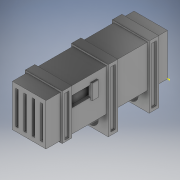
# Autodesk Inventor part: Part1
Saved by Autodesk Inventor 2021 (Build 250183000, 183)
## iProperties
Created: 2021-05-04
Part Number: Part1
Material: Generic
Document SubType Name: Modeling
Designer: AHUJA
Density: 1 g/cm^3
Appearance: Default
Author: AHUJA
Autodesk Inventor part; units mm, degrees
(part 1 of 2)
ref_plane "YZ Plane" through (0, 0, 0) normal (1, 0, 0) x (0, 1, 0)
ref_plane "XZ Plane" through (0, 0, 0) normal (0, 1, 0) x (-1, 0, 0)
sketch "Sketch1" plane through (0, 0, 0) normal (0, 0, 1) x (1, 0, 0)
  line L0 (0, 0) -> (50.8, 0)
  line L1 (50.8, 0) -> (50.8, 63.5)
  line L2 (50.8, 63.5) -> (0, 63.5)
  line L3 (0, 63.5) -> (0, 0)
  dimension "d0" = 63.5
  dimension "d1" = 50.8
  constraints: 8 end point, 2 parallel, 1 horizontal, 1 perpendicular
  measures "d0" distance of L0.end L1.end
  measures "d1" distance of L1.end L2.end
extrude "Extrusion1" add sketch "Sketch1" along normal blind 184.15
sketch "Sketch2" plane through (0, 0, 184.15) normal (0, 0, 1) x (1, 0, 0)
  line L0 (5.021, 56.896) -> (8.763, 56.896)
  line L1 (8.763, 56.896) -> (8.763, 6.604)
  line L2 (8.763, 6.604) -> (5.021, 6.604)
  line L3 (5.021, 6.604) -> (5.021, 56.896)
  line L4 (0, 63.5) -> (0, 0) projected
  line L5 (50.8, 63.5) -> (0, 63.5) projected
  line L6 (17.467, 56.896) -> (21.209, 56.896)
  line L7 (21.209, 56.896) -> (21.209, 6.604)
  line L8 (21.209, 6.604) -> (17.467, 6.604)
  line L9 (17.467, 6.604) -> (17.467, 56.896)
  line L10 (29.913, 56.896) -> (33.655, 56.896)
  line L11 (33.655, 56.896) -> (33.655, 6.604)
  line L12 (33.655, 6.604) -> (29.913, 6.604)
  line L13 (29.913, 6.604) -> (29.913, 56.896)
  line L14 (42.359, 56.896) -> (46.101, 56.896)
  line L15 (46.101, 56.896) -> (46.101, 6.604)
  line L16 (46.101, 6.604) -> (42.359, 6.604)
  line L17 (42.359, 6.604) -> (42.359, 56.896)
  line L18 (50.8, 0) -> (50.8, 63.5) projected
  dimension "d4" = 3.742
  dimension "d5" = 50.292
  dimension "d6" = 5.021
  dimension "d7" = 6.604
  dimension "d8" = 8.704
  dimension "d9" = 6.604
  dimension "d10" = 3.742
  dimension "d11" = 3.742
  dimension "d12" = 8.704
  dimension "d13" = 3.742
  dimension "d16" = 8.704
  constraints: 32 end point, 8 parallel, 4 horizontal, 4 perpendicular
  measures "d4" distance of L0.start L0.end
  measures "d5" distance of L0.end L1.end
  measures "d6" distance between parallel lines of L4 L3
  measures "d7" distance between parallel lines of L5 L0
  measures "d8" distance between parallel lines of L1 L9
  measures "d9" distance between parallel lines of L5 L6
  measures "d10" distance of L6.start L6.end
  measures "d11" distance of L10.start L10.end
  measures "d12" distance between parallel lines of L13 L7
  measures "d13" distance of L14.start L14.end
  measures "d16" distance between parallel lines of L17 L11
extrude "Extrusion2" cut sketch "Sketch2" against normal blind 100
sketch "Sketch3" plane through (0, 0, 0) normal (-1, 0, 0) x (0, 0, 1)
  line L0 (15.895, 66.04) -> (30.358, 66.04)
  line L1 (30.358, 66.04) -> (30.358, -28.667)
  line L2 (30.358, -28.667) -> (15.895, -28.667)
  line L3 (15.895, -28.667) -> (15.895, 66.04)
  line L4 (0, 63.5) -> (0, 0) projected
  line L5 (0, 63.5) -> (184.15, 63.5) projected
  line L6 (77.905, 66.04) -> (92.368, 66.04)
  line L7 (92.368, 66.04) -> (92.368, -28.667)
  line L8 (92.368, -28.667) -> (77.905, -28.667)
  line L9 (77.905, -28.667) -> (77.905, 66.04)
  line L10 (147.737, 66.04) -> (162.2, 66.04)
  line L11 (162.2, 66.04) -> (162.2, -2.54)
  line L12 (162.2, -2.54) -> (147.737, -2.54)
  line L13 (147.737, -2.54) -> (147.737, 66.04)
  dimension "d19" = 94.707
  dimension "d20" = 14.463
  dimension "d21" = 15.895
  dimension "d22" = 2.54
  dimension "d23" = 94.707
  dimension "d24" = 14.463
  dimension "d25" = 68.58
  dimension "d26" = 14.463
  dimension "d27" = 2.54
  dimension "d28" = 2.54
  dimension "d29" = 47.547
  dimension "d30" = 55.369
  constraints: 24 end point, 6 parallel, 3 horizontal, 3 perpendicular
  measures "d19" distance of L0.end L1.end
  measures "d20" distance of L0.start L0.end
  measures "d21" distance between parallel lines of L4 L3
  measures "d22" distance between parallel lines of L5 L0
  measures "d23" distance of L6.end L7.end
  measures "d24" distance of L6.start L6.end
  measures "d25" distance of L10.end L11.end
  measures "d26" distance of L10.start L10.end
  measures "d27" distance between parallel lines of L5 L10
  measures "d28" distance between parallel lines of L5 L6
  measures "d29" distance between parallel lines of L9 L1
  measures "d30" distance between parallel lines of L13 L7
ref_plane "Work Plane1" through (53.34, 0, 0) normal (1, 0, 0) x (0, 0, -1)
extrude "Extrusion3" add sketch "Sketch3" along normal blind 55.88 from surface at -53.34
sketch "Sketch4" plane through (-2.54, -28.667, 30.358) normal (-1, 0, 0) x (0, 0, 1)
  point P0 (-30.358, 28.667)
sketch "Sketch5" plane through (-2.54, -28.667, 30.358) normal (-1, 0, 0) x (0, 0, 1)
  line L0 (-10.738, 90.177) -> (-3.756, 90.177)
  line L1 (-3.756, 90.177) -> (-3.756, 4.938)
  line L2 (-3.756, 4.938) -> (-10.738, 4.938)
  line L3 (-10.738, 4.938) -> (-10.738, 90.177)
  line L4 (-14.463, 94.707) -> (-14.463, 0) projected
  line L5 (51.272, 90.177) -> (58.254, 90.177)
  line L6 (58.254, 90.177) -> (58.254, 4.938)
  line L7 (58.254, 4.938) -> (51.272, 4.938)
  line L8 (51.272, 4.938) -> (51.272, 90.177)
  line L9 (47.547, 94.707) -> (47.547, 0) projected
  line L10 (0, 94.707) -> (-14.463, 94.707) projected
  line L11 (62.01, 94.707) -> (47.547, 94.707) projected
  line L12 (121.666, 90.087) -> (127.547, 90.087)
  line L13 (127.547, 90.087) -> (127.547, 28.667)
  line L14 (127.547, 28.667) -> (121.666, 28.667)
  line L15 (121.666, 28.667) -> (121.666, 90.087)
  line L16 (117.379, 94.707) -> (117.379, 26.127) projected
  point P0 (-30.358, 28.667)
  dimension "d34" = 6.982
  dimension "d35" = 85.239
  dimension "d36" = 3.725
  dimension "d37" = 6.982
  dimension "d38" = 85.239
  dimension "d39" = 3.725
  dimension "d40" = 4.53
  dimension "d41" = 4.53
  dimension "d42" = 61.42
  dimension "d43" = 5.881
  dimension "d44" = 4.287
  constraints: 24 end point, 6 parallel, 3 horizontal, 3 perpendicular
  measures "d34" distance of L0.start L0.end
  measures "d35" distance of L0.end L1.end
  measures "d36" distance between parallel lines of L4 L3
  measures "d37" distance of L5.start L5.end
  measures "d38" distance of L5.end L6.end
  measures "d39" distance between parallel lines of L9 L8
  measures "d40" distance between parallel lines of L10 L0
  measures "d41" distance between parallel lines of L11 L5
  measures "d42" distance of L12.end L13.end
  measures "d43" distance of L12.start L12.end
  measures "d44" distance between parallel lines of L16 L15
extrude "Extrusion4" cut sketch "Sketch5" against normal blind 2.54
sketch "Sketch6" plane through (0, 0, 92.368) normal (-1, 0, 0) x (0, 0, 1)
  line L0 (14.937, 53.681) -> (24.354, 53.681)
  line L1 (24.354, 53.681) -> (24.354, 30.706)
  line L2 (24.354, 30.706) -> (14.937, 30.706)
  line L3 (14.937, 30.706) -> (14.937, 53.681)
  line L4 (0, -28.667) -> (0, 66.04) projected
  line L5 (0, 63.5) -> (55.369, 63.5) projected
  point P0 (-92.368, 0)
  dimension "d48" = 9.417
  dimension "d49" = 14.937
  dimension "d50" = 9.819
  dimension "d51" = 22.975
  constraints: 8 end point, 2 parallel, 1 horizontal, 1 perpendicular
  measures "d48" distance of L0.start L0.end
  measures "d49" distance between parallel lines of L4 L3
  measures "d50" distance between parallel lines of L5 L0
  measures "d51" distance of L2.end L0.start
extrude "Extrusion5" add sketch "Sketch6" along normal blind 1.905
sketch "Sketch7" plane through (0, 0, 92.368) normal (-1, 0, 0) x (0, 0, 1)
  line L0 (24.354, 30.706) -> (24.354, 53.681) projected
  line L1 (24.354, 50.479) -> (55.5483, 50.479)
  line L2 (55.5483, 50.479) -> (55.5483, 34.348)
  line L3 (55.5483, 34.348) -> (24.354, 34.348)
  line L4 (24.354, 34.348) -> (24.354, 50.479)
  line L5 (0, 63.5) -> (55.369, 63.5) projected
  point P0 (-92.368, 0)
  dimension "d54" = 13.021
  dimension "d55" = 16.131
  constraints: 8 end point, 2 parallel, 1 horizontal, 1 perpendicular, 1 point on line
  measures "d54" distance between parallel lines of L5 L1
  measures "d55" distance of L1.end L2.end
extrude "Extrusion6" cut sketch "Sketch7" against normal blind 6.926
sketch "Sketch8" plane through (-1.905, 53.681, 116.722) normal (0, 0, 1) x (1, 0, 0)
  point P0 (1.905, -53.681)
sketch "Sketch9" plane through (-1.905, 53.681, 116.722) normal (0, 0, 1) x (1, 0, 0)
  line L0 (1.905, -19.333) -> (6.926, -19.333) projected
  line L1 (6.926, -19.333) -> (5.021, -19.333)
  line L2 (5.021, -19.333) -> (5.021, -3.202)
  line L3 (5.021, -3.202) -> (6.926, -3.202)
  line L4 (6.926, -3.202) -> (6.926, -19.333)
  point P0 (1.905, -53.681)
  dimension "d58" = 16.131
  dimension "d59" = 1.905
  constraints: 8 end point, 2 parallel, 1 horizontal, 1 perpendicular
  measures "d58" distance of L1.end L2.end
  measures "d59" distance of L0.end L1.end
extrude "Extrusion7" cut sketch "Sketch9" against normal blind 9.417
sketch "Sketch10" plane through (53.34, 66.04, 15.895) normal (0, 0, -1) x (-1, 0, 0)
  circle A0 centre (28.738, -80.425) radius 12.0905
  line L0 (55.88, 0) -> (55.88, -94.707) projected
  line L1 (0, -94.707) -> (55.88, -94.707) projected
  point P0 (53.34, -66.04)
  dimension "d62" = 27.142
  dimension "d63" = 14.282
  dimension "d64" = 24.181
  constraints: 1 centre point
  measures "d62" distance from line of L0 A0.centre
  measures "d63" distance from line of L1 A0.centre
  measures "d64" diameter of A0
sketch "Sketch11" plane through (53.34, 66.04, 77.905) normal (0, 0, -1) x (-1, 0, 0)
  circle A0 centre (27.142, -80.425) radius 12.0905
  line L0 (0, -94.707) -> (55.88, -94.707) projected
  line L1 (0, 0) -> (0, -94.707) projected
  point P0 (53.34, -66.04)
  dimension "d65" = 24.181
  dimension "d66" = 14.282
  dimension "d67" = 27.142
  constraints: 1 centre point
  measures "d65" diameter of A0
  measures "d66" distance from line of L0 A0.centre
  measures "d67" distance from line of L1 A0.centre
extrude "Extrusion8" cut sketch "Sketch10" against normal blind 30
extrude "Extrusion9" cut sketch "Sketch11" against normal blind 30
sketch "Sketch12" plane through (0, 0, 0) normal (0, 0, -1) x (-1, 0, 0)
  line L0 (-25.449, 0) -> (-24.765, 0)
  line L1 (-24.765, 0) -> (-24.765, 0.127)
  line L2 (-24.765, 0.127) -> (-25.449, 0.127)
  line L3 (-25.449, 0.127) -> (-25.449, 0)
  line L4 (0, 63.5) -> (0, 0) projected
  dimension "d72" = 0.127
  dimension "d73" = 0.684
  dimension "d74" = 24.765
  constraints: 8 end point, 2 parallel, 1 horizontal, 1 perpendicular
  measures "d72" distance of L0.end L1.end
  measures "d73" distance of L1.end L2.end
  measures "d74" distance between parallel lines of L4 L1
extrude "Extrusion10" cut sketch "Sketch12" against normal blind 500
sketch "Sketch13" plane through (50.8, 0, 92.368) normal (1, 0, 0) x (0, 0, -1)
  point P0 (92.368, 0)
sketch "Sketch14" plane through (50.8, 0, 92.368) normal (1, 0, 0) x (0, 0, -1)
  line L0 (-55.369, 56.896) -> (-55.369, 6.604) projected
  line L1 (-24.354, 50.479) -> (-24.354, 34.348)
  line L2 (-55.369, 34.348) -> (-55.369, 50.479)
  line L3 (0, 63.5) -> (-55.369, 63.5) projected
  line L4 (-14.937, 53.681) -> (-24.354, 53.681)
  line L5 (-24.354, 53.681) -> (-24.354, 30.706)
  line L6 (-24.354, 30.706) -> (-14.937, 30.706)
  line L7 (-14.937, 30.706) -> (-14.937, 53.681)
  point P0 (92.368, 0)
  point P1 (-24.354, 50.479)
  point P2 (-24.354, 34.348)
  dimension "d77" = 31.015
  dimension "d80" = 9.819
  dimension "d81" = 9.417
  dimension "d82" = 22.975
  constraints: 12 end point, 3 parallel, 1 horizontal, 1 perpendicular, 1 point on line
  measures "d77" distance of L2.end L1.start
  measures "d80" distance between parallel lines of L3 L4
  measures "d81" distance of L4.start L4.end
  measures "d82" distance of L6.end L4.start
extrude "Extrusion11" add sketch "Sketch14" along normal mid plane 5.021
sketch "Sketch15" plane through (50.8, 0, 92.368) normal (1, 0, 0) x (0, 0, -1)
  line L0 (-55.369, 63.5) -> (-55.369, 0) projected
  line L1 (-24.354, 53.681) -> (-24.354, 30.706) projected
  line L2 (-55.369, 50.479) -> (-24.354, 50.479)
  line L3 (-24.354, 50.479) -> (-24.354, 34.348)
  line L4 (-24.354, 34.348) -> (-55.369, 34.348)
  line L5 (-55.369, 34.348) -> (-55.369, 50.479)
  line L6 (0, 63.5) -> (-55.369, 63.5) projected
  point P0 (92.368, 0)
  dimension "d85" = 16.131
  dimension "d86" = 13.021
  constraints: 8 end point, 2 parallel, 2 point on line, 1 horizontal, 1 perpendicular
  measures "d85" distance between parallel lines of L4 L2
  measures "d86" distance between parallel lines of L6 L2
extrude "Extrusion12" cut sketch "Sketch15" against normal blind 5.021
sketch "Sketch16" plane through (50.8, 30.706, 116.722) normal (0, 0, 1) x (1, 0, 0)
  line L0 (0, 3.642) -> (-4.699, 3.642) projected
  line L1 (-4.699, 3.642) -> (-2.794, 3.642)
  line L2 (-2.794, 3.642) -> (-2.794, 19.773)
  line L3 (-2.794, 19.773) -> (-4.699, 19.773)
  line L4 (-4.699, 19.773) -> (-4.699, 3.642)
  point P0 (-50.8, -30.706)
  point P1 (-2.794, 3.642)
  dimension "d89" = 16.131
  dimension "d90" = 1.905
  constraints: 8 end point, 2 parallel, 1 horizontal, 1 perpendicular
  measures "d89" distance of L1.end L2.end
  measures "d90" distance of L2.end L3.end
extrude "Extrusion13" cut sketch "Sketch16" against normal blind 9.417
sketch "Sketch17" plane through (50.8, 0, 92.368) normal (0, -1, 0) x (1, 0, 0)
  line L0 (-40.298, 34.057) -> (-10.502, 34.057)
  line L1 (-10.502, 34.057) -> (-10.502, 27.55)
  line L2 (-10.502, 27.55) -> (-40.298, 27.55)
  line L3 (-40.298, 27.55) -> (-40.298, 34.057)
  line L4 (0, 0) -> (0, 55.369) projected
  line L5 (-50.8, 0) -> (-50.8, 55.369) projected
  line L6 (2.54, 55.369) -> (-53.34, 55.369) projected
  line L7 (-40.298, -35.775) -> (-10.502, -35.775)
  line L8 (-10.502, -35.775) -> (-10.502, -42.282)
  line L9 (-10.502, -42.282) -> (-40.298, -42.282)
  line L10 (-40.298, -42.282) -> (-40.298, -35.775)
  line L11 (0, -62.01) -> (0, -14.463) projected
  line L12 (-50.8, -62.01) -> (-50.8, -14.463) projected
  line L13 (2.54, -14.463) -> (-53.34, -14.463) projected
  point P0 (-50.8, -92.368)
  dimension "d93" = 10.502
  dimension "d94" = 10.502
  dimension "d95" = 6.507
  dimension "d96" = 21.312
  dimension "d97" = 6.507
  dimension "d98" = 10.502
  dimension "d99" = 10.502
  dimension "d100" = 21.312
  constraints: 16 end point, 4 parallel, 2 horizontal, 2 perpendicular
  measures "d93" distance between parallel lines of L4 L1
  measures "d94" distance between parallel lines of L5 L3
  measures "d95" distance between parallel lines of L2 L0
  measures "d96" distance between parallel lines of L0 L6
  measures "d97" distance between parallel lines of L9 L7
  measures "d98" distance between parallel lines of L11 L8
  measures "d99" distance between parallel lines of L12 L10
  measures "d100" distance between parallel lines of L13 L7
extrude "Extrusion14" add sketch "Sketch17" along normal blind 2.54
sketch "Sketch18" plane through (53.34, -2.54, 147.737) normal (1, 0, 0) x (0, 0, -1)
  point P0 (147.737, 2.54)
sketch "Sketch19" plane through (53.34, -2.54, 147.737) normal (1, 0, 0) x (0, 0, -1)
  point P0 (147.737, 2.54)
sketch "Sketch20" plane through (53.34, -2.54, 147.737) normal (1, 0, 0) x (0, 0, -1)
  line L0 (-10.168, 63.96) -> (-4.287, 63.96)
  line L1 (-4.287, 63.96) -> (-4.287, 2.54)
  line L2 (-4.287, 2.54) -> (-10.168, 2.54)
  line L3 (-10.168, 2.54) -> (-10.168, 63.96)
  line L4 (-14.463, 68.58) -> (0, 68.58) projected
  line L5 (-14.463, 0) -> (-14.463, 68.58) projected
  line L6 (59.094, 63.642) -> (66.076, 63.642)
  line L7 (66.076, 63.642) -> (66.076, -21.597)
  line L8 (66.076, -21.597) -> (59.094, -21.597)
  line L9 (59.094, -21.597) -> (59.094, 63.642)
  line L10 (55.369, 68.58) -> (69.832, 68.58) projected
  line L11 (55.369, -26.127) -> (55.369, 68.58) projected
  line L12 (121.104, 63.642) -> (128.086, 63.642)
  line L13 (128.086, 63.642) -> (128.086, -21.597)
  line L14 (128.086, -21.597) -> (121.104, -21.597)
  line L15 (121.104, -21.597) -> (121.104, 63.642)
  line L16 (117.379, 68.58) -> (131.842, 68.58) projected
  line L17 (117.379, -26.127) -> (117.379, 68.58) projected
  point P0 (147.737, 2.54)
  dimension "d103" = 5.881
  dimension "d104" = 61.42
  dimension "d105" = 4.62
  dimension "d106" = 4.295
  dimension "d107" = 6.982
  dimension "d108" = 85.239
  dimension "d109" = 4.938
  dimension "d110" = 3.725
  dimension "d111" = 6.982
  dimension "d112" = 85.239
  dimension "d113" = 4.938
  dimension "d114" = 3.725
  constraints: 24 end point, 6 parallel, 3 horizontal, 3 perpendicular
  measures "d103" distance of L0.start L0.end
  measures "d104" distance of L0.end L1.end
  measures "d105" distance between parallel lines of L4 L0
  measures "d106" distance between parallel lines of L5 L3
  measures "d107" distance of L6.start L6.end
  measures "d108" distance of L6.end L7.end
  measures "d109" distance between parallel lines of L10 L6
  measures "d110" distance between parallel lines of L11 L9
  measures "d111" distance of L12.start L12.end
  measures "d112" distance of L12.end L14.start
  measures "d113" distance between parallel lines of L12 L16
  measures "d114" distance between parallel lines of L17 L15
extrude "Extrusion15" cut sketch "Sketch20" against normal blind 2.54
sketch "Sketch21" plane through (0, 0, 0) normal (0, 0, -1) x (-1, 0, 0)
  line L0 (-20.0547, 62.7614) -> (-0.3775, 62.7614) construction
  line L1 (-0.3775, 62.7614) -> (-0.3775, 56.8982) construction
  line L2 (-0.3775, 56.8982) -> (-20.0547, 56.8982) construction
  line L3 (-20.0547, 56.8982) -> (-20.0547, 62.7614) construction
  spline S0 degree 2 poles (-17.5491, 61.6438) (-16.5595, 62.6455) (-16.2827, 62.6455) knots 0 0 0 1 1 1
  spline S1 degree 2 poles (-16.2827, 62.6455) (-16.1668, 62.6455) (-16.1668, 62.5365) knots 0 0 0 1 1 1
  spline S2 degree 2 poles (-16.1668, 62.5365) (-16.1668, 62.4344) (-16.2498, 62.3099) knots 0 0 0 1 1 1
  spline S3 degree 2 poles (-16.2498, 62.3099) (-16.3121, 62.2216) (-16.9972, 61.5036) knots 0 0 0 1 1 1
  spline S4 degree 2 poles (-16.9972, 61.5036) (-17.5682, 60.8704) (-17.5682, 60.7597) knots 0 0 0 1 1 1
  spline S5 degree 2 poles (-17.5682, 60.7597) (-17.5682, 60.7216) (-17.4574, 60.713) (-17.4574, 60.7009) knots 0 0 0 1 2 2 2
  spline S6 degree 2 poles (-17.4574, 60.7009) (-17.4574, 60.6611) (-17.5439, 60.6611) knots 0 0 0 1 1 1
  spline S7 degree 2 poles (-17.5439, 60.6611) (-17.6668, 60.6611) (-17.6668, 60.777) knots 0 0 0 1 1 1
  spline S8 degree 2 poles (-17.6668, 60.777) (-17.6668, 60.9915) (-17.1339, 61.5849) knots 0 0 0 1 1 1
  spline S9 degree 2 poles (-17.1339, 61.5849) (-16.9471, 61.7943) (-16.4263, 62.3168) knots 0 0 0 1 1 1
  spline S10 degree 2 poles (-16.4263, 62.3168) (-16.2481, 62.4933) (-16.2481, 62.5642) knots 0 0 0 1 1 1
  spline S11 degree 2 poles (-16.2481, 62.5642) (-16.2481, 62.5919) (-16.2758, 62.5919) knots 0 0 0 1 1 1
  spline S12 degree 2 poles (-16.2758, 62.5919) (-16.3744, 62.5919) (-16.8311, 62.213) knots 0 0 0 1 1 1
  spline S13 degree 2 poles (-16.8311, 62.213) (-17.1962, 61.9085) (-17.3761, 61.7285) knots 0 0 0 1 1 1
  spline S14 degree 2 poles (-17.3761, 61.7285) (-17.5491, 61.5555) (-17.8311, 61.2407) knots 0 0 0 1 1 1
  spline S15 degree 2 poles (-17.8311, 61.2407) (-18.3381, 60.6715) (-18.3536, 60.6715) knots 0 0 0 1 1 1
  spline S16 degree 2 poles (-18.3536, 60.6715) (-18.3744, 60.6715) (-18.4332, 60.7251) (-18.4332, 60.7476) knots 0 0 0 1 2 2 2
  spline S17 degree 2 poles (-18.4332, 60.7476) (-18.4332, 60.8029) (-17.2204, 62.2355) (-17.2204, 62.3497) knots 0 0 0 1 2 2 2
  spline S18 degree 2 poles (-17.2204, 62.3497) (-17.2204, 62.3791) (-17.2481, 62.3791) knots 0 0 0 1 1 1
  spline S19 degree 2 poles (-17.2481, 62.3791) (-17.3225, 62.3791) (-17.6253, 62.1507) knots 0 0 0 1 1 1
  spline S20 degree 2 poles (-17.6253, 62.1507) (-17.9055, 61.9396) (-18.2412, 61.6195) knots 0 0 0 1 1 1
  line L4 (-18.2412, 61.6195) -> (-18.819, 61.0469)
  line L5 (-18.819, 61.0469) -> (-19.0215, 60.8289)
  spline S21 degree 2 poles (-19.0215, 60.8289) (-19.191, 60.6455) (-19.2048, 60.6455) knots 0 0 0 1 1 1
  spline S22 degree 2 poles (-19.2048, 60.6455) (-19.2273, 60.6455) (-19.2619, 60.668) knots 0 0 0 1 1 1
  spline S23 degree 2 poles (-19.2619, 60.668) (-19.3, 60.6922) (-19.3, 60.7147) knots 0 0 0 1 1 1
  spline S24 degree 2 poles (-19.3, 60.7147) (-19.3, 60.7614) (-18.9419, 61.1628) knots 0 0 0 1 1 1
  line L6 (-18.9419, 61.1628) -> (-18.274, 61.9137)
  spline S25 degree 2 poles (-18.274, 61.9137) (-17.9142, 62.3358) (-17.9142, 62.4362) knots 0 0 0 1 1 1
  spline S26 degree 2 poles (-17.9142, 62.4362) (-17.9142, 62.4725) (-17.9505, 62.4725) knots 0 0 0 1 1 1
  spline S27 degree 2 poles (-17.9505, 62.4725) (-18.0543, 62.4725) (-18.3796, 62.2078) knots 0 0 0 1 1 1
  spline S28 degree 2 poles (-18.3796, 62.2078) (-18.6235, 62.0106) (-19.0751, 61.5088) knots 0 0 0 1 1 1
  spline S29 degree 2 poles (-19.0751, 61.5088) (-19.1045, 61.4777) (-19.1218, 61.4777) knots 0 0 0 1 1 1
  spline S30 degree 2 poles (-19.1218, 61.4777) (-19.1529, 61.4777) (-19.1529, 61.5019) knots 0 0 0 1 1 1
  spline S31 degree 2 poles (-19.1529, 61.5019) (-19.1529, 61.5382) (-18.9038, 61.8254) knots 0 0 0 1 1 1
  spline S32 degree 2 poles (-18.9038, 61.8254) (-18.7239, 62.0279) (-18.4522, 62.2545) knots 0 0 0 1 1 1
  spline S33 degree 2 poles (-18.4522, 62.2545) (-18.0993, 62.5452) (-17.9419, 62.5452) knots 0 0 0 1 1 1
  spline S34 degree 2 poles (-17.9419, 62.5452) (-17.8363, 62.5452) (-17.8363, 62.4292) knots 0 0 0 1 1 1
  spline S35 degree 2 poles (-17.8363, 62.4292) (-17.8363, 62.2355) (-18.3502, 61.6074) knots 0 0 0 1 1 1
  spline S36 degree 2 poles (-18.3502, 61.6074) (-17.473, 62.4431) (-17.2481, 62.4431) knots 0 0 0 1 1 1
  spline S37 degree 2 poles (-17.2481, 62.4431) (-17.1426, 62.4431) (-17.1426, 62.3341) knots 0 0 0 1 1 1
  spline S38 degree 2 poles (-17.1426, 62.3341) (-17.1426, 62.1628) (-17.5491, 61.6438) knots 0 0 0 1 1 1
  spline S39 degree 2 poles (-16.5682, 60.758) (-16.5682, 60.7199) (-16.4851, 60.7199) knots 0 0 0 1 1 1
  spline S40 degree 2 poles (-16.4851, 60.7199) (-16.4661, 60.7199) (-16.4661, 60.6957) knots 0 0 0 1 1 1
  spline S41 degree 2 poles (-16.4661, 60.6957) (-16.4661, 60.668) (-16.5612, 60.668) knots 0 0 0 1 1 1
  spline S42 degree 2 poles (-16.5612, 60.668) (-16.6685, 60.668) (-16.6685, 60.7701) knots 0 0 0 1 1 1
  spline S43 degree 2 poles (-16.6685, 60.7701) (-16.6685, 60.8912) (-16.3502, 61.2718) knots 0 0 0 1 1 1
  line L7 (-16.3502, 61.2718) -> (-16.7394, 60.9535)
  spline S44 degree 2 poles (-16.7394, 60.9535) (-17.0855, 60.6715) (-17.2412, 60.6715) knots 0 0 0 1 1 1
  spline S45 degree 2 poles (-17.2412, 60.6715) (-17.2585, 60.6715) (-17.2585, 60.6905) knots 0 0 0 1 1 1
  spline S46 degree 2 poles (-17.2585, 60.6905) (-17.2585, 60.7182) (-17.2291, 60.7234) knots 0 0 0 1 1 1
  spline S47 degree 2 poles (-17.2291, 60.7234) (-17.1408, 60.7407) (-17.0664, 60.7822) knots 0 0 0 1 1 1
  spline S48 degree 2 poles (-17.0664, 60.7822) (-16.973, 60.8324) (-16.672, 61.0711) knots 0 0 0 1 1 1
  line L8 (-16.672, 61.0711) -> (-16.236, 61.4362)
  spline S49 degree 2 poles (-16.236, 61.4362) (-16.2066, 61.4465) (-16.1581, 61.4465) knots 0 0 0 1 1 1
  spline S50 degree 2 poles (-16.1581, 61.4465) (-16.1097, 61.4465) (-16.1097, 61.3912) knots 0 0 0 1 1 1
  spline S51 degree 2 poles (-16.1097, 61.3912) (-16.1097, 61.3306) (-16.5682, 60.8047) (-16.5682, 60.758) knots 0 0 0 1 2 2 2
  spline S52 degree 2 poles (-15.9384, 61.7458) (-16.0076, 61.7458) (-16.0076, 61.8151) knots 0 0 0 1 1 1
  spline S53 degree 2 poles (-16.0076, 61.8151) (-16.0076, 61.8739) (-15.9384, 61.9206) knots 0 0 0 1 1 1
  spline S54 degree 2 poles (-15.9384, 61.9206) (-15.8744, 61.9638) (-15.8121, 61.9638) knots 0 0 0 1 1 1
  spline S55 degree 2 poles (-15.8121, 61.9638) (-15.7377, 61.9638) (-15.7377, 61.8825) knots 0 0 0 1 1 1
  spline S56 degree 2 poles (-15.7377, 61.8825) (-15.7377, 61.8237) (-15.8121, 61.7822) knots 0 0 0 1 1 1
  spline S57 degree 2 poles (-15.8121, 61.7822) (-15.8761, 61.7458) (-15.9384, 61.7458) knots 0 0 0 1 1 1
  line L9 (-15.537, 61.3306) -> (-15.9194, 61.0088)
  line L10 (-15.9194, 61.0088) -> (-16.1824, 60.8029)
  spline S58 degree 2 poles (-16.1824, 60.8029) (-16.3692, 60.6715) (-16.4886, 60.6715) knots 0 0 0 1 1 1
  spline S59 degree 2 poles (-16.4886, 60.6715) (-16.5059, 60.6715) (-16.5059, 60.6905) knots 0 0 0 1 1 1
  spline S60 degree 2 poles (-16.5059, 60.6905) (-16.5059, 60.7164) (-16.4765, 60.7234) knots 0 0 0 1 1 1
  spline S61 degree 2 poles (-16.4765, 60.7234) (-16.2896, 60.7683) (-15.9678, 61.0348) knots 0 0 0 1 1 1
  line L11 (-15.9678, 61.0348) -> (-15.5612, 61.3739)
  spline S62 degree 2 poles (-15.5612, 61.3739) (-15.4211, 61.4915) (-15.1097, 61.8375) knots 0 0 0 1 1 1
  line L12 (-15.1097, 61.8375) -> (-14.71, 62.2943)
  spline S63 degree 2 poles (-14.71, 62.2943) (-14.6149, 62.4067) (-14.5768, 62.4067) knots 0 0 0 1 1 1
  spline S64 degree 2 poles (-14.5768, 62.4067) (-14.5266, 62.4067) (-14.5266, 62.3566) knots 0 0 0 1 1 1
  spline S65 degree 2 poles (-14.5266, 62.3566) (-14.5266, 62.2943) (-14.6495, 62.142) knots 0 0 0 1 1 1
  line L13 (-14.6495, 62.142) -> (-14.8259, 61.9413)
  line L14 (-14.8259, 61.9413) -> (-15.3952, 61.2856)
  spline S66 degree 2 poles (-15.3952, 61.2856) (-15.1858, 61.4362) (-15.0872, 61.4362) knots 0 0 0 1 1 1
  spline S67 degree 2 poles (-15.0872, 61.4362) (-14.9713, 61.4362) (-14.9713, 61.322) knots 0 0 0 1 1 1
  spline S68 degree 2 poles (-14.9713, 61.322) (-14.9713, 61.1939) (-15.1962, 61.1022) knots 0 0 0 1 1 1
  spline S69 degree 2 poles (-15.1962, 61.1022) (-15.3796, 61.0279) (-15.537, 61.0261) knots 0 0 0 1 1 1
  spline S70 degree 2 poles (-15.537, 61.0261) (-15.4868, 60.905) (-15.4055, 60.751) knots 0 0 0 1 1 1
  spline S71 degree 2 poles (-15.4055, 60.751) (-15.3779, 60.7182) (-15.3173, 60.7182) knots 0 0 0 1 1 1
  spline S72 degree 2 poles (-15.3173, 60.7182) (-15.2965, 60.7182) (-15.2965, 60.6957) knots 0 0 0 1 1 1
  spline S73 degree 2 poles (-15.2965, 60.6957) (-15.2965, 60.6645) (-15.4073, 60.6645) knots 0 0 0 1 1 1
  spline S74 degree 2 poles (-15.4073, 60.6645) (-15.4626, 60.6645) (-15.5007, 60.6922) knots 0 0 0 1 1 1
  spline S75 degree 2 poles (-15.5007, 60.6922) (-15.5353, 60.7164) (-15.6564, 60.9742) knots 0 0 0 1 1 1
  line L15 (-15.6564, 60.9742) -> (-15.8, 60.8029)
  spline S76 degree 2 poles (-15.8, 60.8029) (-15.9194, 60.6628) (-15.9436, 60.6628) knots 0 0 0 1 1 1
  spline S77 degree 2 poles (-15.9436, 60.6628) (-16.0042, 60.6628) (-16.0042, 60.7337) knots 0 0 0 1 1 1
  spline S78 degree 2 poles (-16.0042, 60.7337) (-16.0042, 60.7753) (-15.7792, 61.0469) knots 0 0 0 1 1 1
  line L16 (-15.7792, 61.0469) -> (-15.537, 61.3306)
  spline S79 degree 2 poles (-15.5803, 61.059) (-15.3675, 61.0867) (-15.0907, 61.2666) (-15.0907, 61.3306) knots 0 0 0 1 2 2 2
  spline S80 degree 2 poles (-15.0907, 61.3306) (-15.0907, 61.3635) (-15.1322, 61.3635) knots 0 0 0 1 1 1
  spline S81 degree 2 poles (-15.1322, 61.3635) (-15.2879, 61.3635) (-15.5803, 61.059) knots 0 0 0 1 1 1
  spline S82 degree 2 poles (-14.7931, 60.9725) (-15.1754, 60.6715) (-15.319, 60.6715) knots 0 0 0 1 1 1
  spline S83 degree 2 poles (-15.319, 60.6715) (-15.3363, 60.6715) (-15.3363, 60.6905) knots 0 0 0 1 1 1
  spline S84 degree 2 poles (-15.3363, 60.6905) (-15.3363, 60.7182) (-15.3017, 60.7234) knots 0 0 0 1 1 1
  spline S85 degree 2 poles (-15.3017, 60.7234) (-15.1685, 60.7441) (-14.9298, 60.931) knots 0 0 0 1 1 1
  line L17 (-14.9298, 60.931) -> (-14.7464, 61.0746)
  line L18 (-14.7464, 61.0746) -> (-14.4505, 61.3099)
  spline S86 degree 2 poles (-14.4505, 61.3099) (-14.2481, 61.45) (-14.1028, 61.45) knots 0 0 0 1 1 1
  spline S87 degree 2 poles (-14.1028, 61.45) (-13.9955, 61.45) (-13.9834, 61.3427) knots 0 0 0 1 1 1
  spline S88 degree 2 poles (-13.9834, 61.3427) (-13.928, 61.3964) (-13.9055, 61.3964) knots 0 0 0 1 1 1
  spline S89 degree 2 poles (-13.9055, 61.3964) (-13.8588, 61.3964) (-13.8588, 61.3566) knots 0 0 0 1 1 1
  spline S90 degree 2 poles (-13.8588, 61.3566) (-13.8588, 61.3064) (-14.2965, 60.796) (-14.2965, 60.7528) knots 0 0 0 1 2 2 2
  spline S91 degree 2 poles (-14.2965, 60.7528) (-14.2965, 60.7234) (-14.2048, 60.7199) (-14.2048, 60.6974) knots 0 0 0 1 2 2 2
  spline S92 degree 2 poles (-14.2048, 60.6974) (-14.2048, 60.668) (-14.3, 60.668) knots 0 0 0 1 1 1
  spline S93 degree 2 poles (-14.3, 60.668) (-14.3952, 60.668) (-14.3952, 60.7528) knots 0 0 0 1 1 1
  spline S94 degree 2 poles (-14.3952, 60.7528) (-14.3952, 60.8202) (-14.319, 60.9431) knots 0 0 0 1 1 1
  line L19 (-14.319, 60.9431) -> (-14.4955, 60.7926)
  spline S95 degree 2 poles (-14.4955, 60.7926) (-14.6253, 60.6957) (-14.7031, 60.6957) knots 0 0 0 1 1 1
  spline S96 degree 2 poles (-14.7031, 60.6957) (-14.8259, 60.6957) (-14.8259, 60.8202) knots 0 0 0 1 1 1
  spline S97 degree 2 poles (-14.8259, 60.8202) (-14.8259, 60.8894) (-14.7931, 60.9725) knots 0 0 0 1 1 1
  spline S98 degree 2 poles (-14.0837, 61.3912) (-14.1685, 61.3912) (-14.6962, 60.8877) (-14.6962, 60.8029) knots 0 0 0 1 2 2 2
  spline S99 degree 2 poles (-14.6962, 60.8029) (-14.6962, 60.7649) (-14.6599, 60.7649) knots 0 0 0 1 1 1
  spline S100 degree 2 poles (-14.6599, 60.7649) (-14.5768, 60.7649) (-14.0422, 61.258) (-14.0422, 61.3445) knots 0 0 0 1 2 2 2
  spline S101 degree 2 poles (-14.0422, 61.3445) (-14.0422, 61.3912) (-14.0837, 61.3912) knots 0 0 0 1 1 1
  spline S102 degree 2 poles (-13.7758, 60.9154) (-14.0734, 60.6715) (-14.2273, 60.6715) knots 0 0 0 1 1 1
  spline S103 degree 2 poles (-14.2273, 60.6715) (-14.2446, 60.6715) (-14.2446, 60.6888) knots 0 0 0 1 1 1
  spline S104 degree 2 poles (-14.2446, 60.6888) (-14.2446, 60.7164) (-14.2152, 60.7234) knots 0 0 0 1 1 1
  spline S105 degree 2 poles (-14.2152, 60.7234) (-14.1633, 60.7355) (-14.0526, 60.7804) knots 0 0 0 1 1 1
  spline S106 degree 2 poles (-14.0526, 60.7804) (-13.9505, 60.8358) (-13.5301, 61.1853) knots 0 0 0 1 1 1
  spline S107 degree 2 poles (-13.5301, 61.1853) (-13.1322, 61.5157) (-13.1218, 61.5157) knots 0 0 0 1 1 1
  spline S108 degree 2 poles (-13.1218, 61.5157) (-13.0889, 61.5157) (-13.0249, 61.4586) (-13.0249, 61.4258) knots 0 0 0 1 2 2 2
  spline S109 degree 2 poles (-13.0249, 61.4258) (-13.0249, 61.322) (-13.1875, 61.059) knots 0 0 0 1 1 1
  spline S110 degree 2 poles (-13.1875, 61.059) (-13.3294, 60.8324) (-13.4349, 60.7199) knots 0 0 0 1 1 1
  spline S111 degree 2 poles (-13.4349, 60.7199) (-13.3727, 60.7199) (-13.3727, 60.6974) knots 0 0 0 1 1 1
  spline S112 degree 2 poles (-13.3727, 60.6974) (-13.3727, 60.668) (-13.4332, 60.668) knots 0 0 0 1 1 1
  spline S113 degree 2 poles (-13.4332, 60.668) (-13.4488, 60.668) (-13.5093, 60.6784) (-13.5266, 60.6784) knots 0 0 0 1 2 2 2
  spline S114 degree 2 poles (-13.5266, 60.6784) (-13.537, 60.6784) (-13.5837, 60.6697) (-13.5941, 60.6697) knots 0 0 0 1 2 2 2
  spline S115 degree 2 poles (-13.5941, 60.6697) (-13.7758, 60.6697) (-13.7758, 60.9154) knots 0 0 0 1 1 1
  spline S116 degree 2 poles (-13.5491, 60.7891) (-13.4488, 60.8721) (-13.3294, 61.0763) knots 0 0 0 1 1 1
  spline S117 degree 2 poles (-13.3294, 61.0763) (-13.2187, 61.2649) (-13.1737, 61.4102) knots 0 0 0 1 1 1
  line L20 (-13.1737, 61.4102) -> (-13.6841, 60.995)
  spline S118 degree 2 poles (-13.6841, 60.995) (-13.6322, 60.9863) (-13.5958, 60.9119) knots 0 0 0 1 1 1
  line L21 (-13.5958, 60.9119) -> (-13.5491, 60.7891)
  line L22 (-13.5889, 60.7458) -> (-13.6287, 60.86)
  spline S119 degree 2 poles (-13.6287, 60.86) (-13.6616, 60.9431) (-13.691, 60.9431) knots 0 0 0 1 1 1
  spline S120 degree 2 poles (-13.691, 60.9431) (-13.7221, 60.9431) (-13.7221, 60.8946) knots 0 0 0 1 1 1
  spline S121 degree 2 poles (-13.7221, 60.8946) (-13.7221, 60.8445) (-13.6945, 60.7926) knots 0 0 0 1 1 1
  spline S122 degree 2 poles (-13.6945, 60.7926) (-13.6616, 60.7337) (-13.6166, 60.7337) knots 0 0 0 1 1 1
  spline S123 degree 2 poles (-13.6166, 60.7337) (-13.5993, 60.7337) (-13.5889, 60.7458) knots 0 0 0 1 1 1
  spline S124 degree 2 poles (-12.8692, 60.9725) (-13.2516, 60.6715) (-13.3952, 60.6715) knots 0 0 0 1 1 1
  spline S125 degree 2 poles (-13.3952, 60.6715) (-13.4125, 60.6715) (-13.4125, 60.6905) knots 0 0 0 1 1 1
  spline S126 degree 2 poles (-13.4125, 60.6905) (-13.4125, 60.7182) (-13.3779, 60.7234) knots 0 0 0 1 1 1
  spline S127 degree 2 poles (-13.3779, 60.7234) (-13.2446, 60.7441) (-13.0059, 60.931) knots 0 0 0 1 1 1
  line L23 (-13.0059, 60.931) -> (-12.8225, 61.0746)
  line L24 (-12.8225, 61.0746) -> (-12.5266, 61.3099)
  spline S128 degree 2 poles (-12.5266, 61.3099) (-12.3242, 61.45) (-12.1789, 61.45) knots 0 0 0 1 1 1
  spline S129 degree 2 poles (-12.1789, 61.45) (-12.0716, 61.45) (-12.0595, 61.3427) knots 0 0 0 1 1 1
  spline S130 degree 2 poles (-12.0595, 61.3427) (-12.0042, 61.3964) (-11.9817, 61.3964) knots 0 0 0 1 1 1
  spline S131 degree 2 poles (-11.9817, 61.3964) (-11.9349, 61.3964) (-11.9349, 61.3566) knots 0 0 0 1 1 1
  spline S132 degree 2 poles (-11.9349, 61.3566) (-11.9349, 61.3064) (-12.3727, 60.796) (-12.3727, 60.7528) knots 0 0 0 1 2 2 2
  spline S133 degree 2 poles (-12.3727, 60.7528) (-12.3727, 60.7234) (-12.281, 60.7199) (-12.281, 60.6974) knots 0 0 0 1 2 2 2
  spline S134 degree 2 poles (-12.281, 60.6974) (-12.281, 60.668) (-12.3761, 60.668) knots 0 0 0 1 1 1
  spline S135 degree 2 poles (-12.3761, 60.668) (-12.4713, 60.668) (-12.4713, 60.7528) knots 0 0 0 1 1 1
  spline S136 degree 2 poles (-12.4713, 60.7528) (-12.4713, 60.8202) (-12.3952, 60.9431) knots 0 0 0 1 1 1
  line L25 (-12.3952, 60.9431) -> (-12.5716, 60.7926)
  spline S137 degree 2 poles (-12.5716, 60.7926) (-12.7014, 60.6957) (-12.7792, 60.6957) knots 0 0 0 1 1 1
  spline S138 degree 2 poles (-12.7792, 60.6957) (-12.9021, 60.6957) (-12.9021, 60.8202) knots 0 0 0 1 1 1
  spline S139 degree 2 poles (-12.9021, 60.8202) (-12.9021, 60.8894) (-12.8692, 60.9725) knots 0 0 0 1 1 1
  spline S140 degree 2 poles (-12.1599, 61.3912) (-12.2446, 61.3912) (-12.7723, 60.8877) (-12.7723, 60.8029) knots 0 0 0 1 2 2 2
  spline S141 degree 2 poles (-12.7723, 60.8029) (-12.7723, 60.7649) (-12.736, 60.7649) knots 0 0 0 1 1 1
  spline S142 degree 2 poles (-12.736, 60.7649) (-12.6529, 60.7649) (-12.1183, 61.258) (-12.1183, 61.3445) knots 0 0 0 1 2 2 2
  spline S143 degree 2 poles (-12.1183, 61.3445) (-12.1183, 61.3912) (-12.1599, 61.3912) knots 0 0 0 1 1 1
  line L26 (-9.0941, 61.495) -> (-8.9644, 61.495)
  spline S144 degree 2 poles (-8.9644, 61.495) (-8.8692, 61.4846) (-8.8692, 61.4362) knots 0 0 0 1 1 1
  spline S145 degree 2 poles (-8.8692, 61.4362) (-8.8692, 61.405) (-8.9384, 61.405) knots 0 0 0 1 1 1
  line L27 (-8.9384, 61.405) -> (-9.0301, 61.4102)
  line L28 (-9.0301, 61.4102) -> (-9.1651, 61.4085)
  line L29 (-9.1651, 61.4085) -> (-9.4557, 61.04)
  spline S146 degree 2 poles (-9.4557, 61.04) (-9.7516, 60.6715) (-9.7827, 60.6715) knots 0 0 0 1 1 1
  spline S147 degree 2 poles (-9.7827, 60.6715) (-9.8104, 60.6715) (-9.8329, 60.713) knots 0 0 0 1 1 1
  spline S148 degree 2 poles (-9.8329, 60.713) (-9.8554, 60.7476) (-9.8554, 60.777) knots 0 0 0 1 1 1
  spline S149 degree 2 poles (-9.8554, 60.777) (-9.8554, 60.822) (-9.3692, 61.4085) knots 0 0 0 1 1 1
  line L30 (-9.3692, 61.4085) -> (-9.4799, 61.4085)
  spline S150 degree 2 poles (-9.4799, 61.4085) (-9.7135, 61.4067) (-10.1737, 61.3843) knots 0 0 0 1 1 1
  line L31 (-10.1737, 61.3843) -> (-10.6547, 60.9708)
  line L32 (-10.6547, 60.9708) -> (-10.8433, 60.8029)
  spline S151 degree 2 poles (-10.8433, 60.8029) (-10.9938, 60.6715) (-11.0266, 60.6715) knots 0 0 0 1 1 1
  spline S152 degree 2 poles (-11.0266, 60.6715) (-11.0664, 60.6715) (-11.0664, 60.713) knots 0 0 0 1 1 1
  spline S153 degree 2 poles (-11.0664, 60.713) (-11.0664, 60.7649) (-10.6547, 61.1092) knots 0 0 0 1 1 1
  line L33 (-10.6547, 61.1092) -> (-10.3277, 61.3808)
  spline S154 degree 2 poles (-10.3277, 61.3808) (-10.9817, 61.3497) (-11.0024, 61.3133) knots 0 0 0 1 1 1
  line L34 (-11.0024, 61.3133) -> (-11.0024, 61.3116)
  spline S155 degree 2 poles (-11.0024, 61.3116) (-11.0024, 61.2839) (-10.7983, 61.2839) knots 0 0 0 1 1 1
  line L35 (-10.7983, 61.2839) -> (-10.608, 61.2874)
  spline S156 degree 2 poles (-10.608, 61.2874) (-10.5699, 61.2874) (-10.5699, 61.2701) knots 0 0 0 1 1 1
  spline S157 degree 2 poles (-10.5699, 61.2701) (-10.5699, 61.2303) (-10.8813, 61.2303) knots 0 0 0 1 1 1
  spline S158 degree 2 poles (-10.8813, 61.2303) (-11.146, 61.2303) (-11.146, 61.2977) knots 0 0 0 1 1 1
  spline S159 degree 2 poles (-11.146, 61.2977) (-11.146, 61.3843) (-10.9886, 61.4171) knots 0 0 0 1 1 1
  spline S160 degree 2 poles (-10.9886, 61.4171) (-10.9453, 61.4258) (-10.7689, 61.4379) knots 0 0 0 1 1 1
  line L36 (-10.7689, 61.4379) -> (-10.2135, 61.4742)
  spline S161 degree 2 poles (-10.2135, 61.4742) (-9.8761, 61.7528) (-9.2498, 62.1974) knots 0 0 0 1 1 1
  spline S162 degree 2 poles (-9.2498, 62.1974) (-8.4522, 62.7614) (-8.2983, 62.7614) knots 0 0 0 1 1 1
  spline S163 degree 2 poles (-8.2983, 62.7614) (-8.2204, 62.7614) (-8.2204, 62.6611) knots 0 0 0 1 1 1
  spline S164 degree 2 poles (-8.2204, 62.6611) (-8.2204, 62.5763) (-8.4211, 62.3272) knots 0 0 0 1 1 1
  line L37 (-8.4211, 62.3272) -> (-9.0941, 61.495)
  line L38 (-9.2983, 61.495) -> (-8.6304, 62.3064)
  line L39 (-8.6304, 62.3064) -> (-8.5059, 62.4586)
  spline S165 degree 2 poles (-8.5059, 62.4586) (-8.4263, 62.559) (-8.4003, 62.6144) knots 0 0 0 1 1 1
  line L40 (-8.4003, 62.6144) -> (-8.3986, 62.6195)
  spline S166 degree 2 poles (-8.3986, 62.6195) (-8.3986, 62.6351) (-8.4125, 62.6351) knots 0 0 0 1 1 1
  spline S167 degree 2 poles (-8.4125, 62.6351) (-8.4799, 62.6351) (-9.2619, 62.0642) knots 0 0 0 1 1 1
  line L41 (-9.2619, 62.0642) -> (-10.0457, 61.4811)
  line L42 (-10.0457, 61.4811) -> (-9.2983, 61.495)
  line L43 (-8.7048, 61.0694) -> (-9.0024, 60.8358)
  spline S168 degree 2 poles (-9.0024, 60.8358) (-9.2343, 60.6715) (-9.3554, 60.6715) knots 0 0 0 1 1 1
  spline S169 degree 2 poles (-9.3554, 60.6715) (-9.3727, 60.6715) (-9.3727, 60.6888) knots 0 0 0 1 1 1
  spline S170 degree 2 poles (-9.3727, 60.6888) (-9.3727, 60.7164) (-9.3381, 60.7234) knots 0 0 0 1 1 1
  spline S171 degree 2 poles (-9.3381, 60.7234) (-9.2048, 60.7493) (-8.9782, 60.9206) knots 0 0 0 1 1 1
  line L44 (-8.9782, 60.9206) -> (-8.582, 61.2372)
  spline S172 degree 2 poles (-8.582, 61.2372) (-8.2567, 61.5036) (-8.082, 61.5036) knots 0 0 0 1 1 1
  spline S173 degree 2 poles (-8.082, 61.5036) (-7.9886, 61.5036) (-7.9886, 61.4327) knots 0 0 0 1 1 1
  spline S174 degree 2 poles (-7.9886, 61.4327) (-7.9574, 61.4327) (-7.9574, 61.405) knots 0 0 0 1 1 1
  spline S175 degree 2 poles (-7.9574, 61.405) (-7.9574, 61.3808) (-7.992, 61.3791) knots 0 0 0 1 1 1
  spline S176 degree 2 poles (-7.992, 61.3791) (-8.0215, 61.277) (-8.0993, 61.1766) knots 0 0 0 1 1 1
  spline S177 degree 2 poles (-8.0993, 61.1766) (-8.1945, 61.0573) (-8.281, 61.0573) knots 0 0 0 1 1 1
  spline S178 degree 2 poles (-8.281, 61.0573) (-8.3329, 61.0573) (-8.3329, 61.104) knots 0 0 0 1 1 1
  spline S179 degree 2 poles (-8.3329, 61.104) (-8.3329, 61.1715) (-8.2221, 61.2787) knots 0 0 0 1 1 1
  spline S180 degree 2 poles (-8.2221, 61.2787) (-8.1235, 61.3739) (-8.0457, 61.4067) knots 0 0 0 1 1 1
  line L45 (-8.0457, 61.4067) -> (-8.0422, 61.4223)
  spline S181 degree 2 poles (-8.0422, 61.4223) (-8.0422, 61.4431) (-8.063, 61.4431) knots 0 0 0 1 1 1
  spline S182 degree 2 poles (-8.063, 61.4431) (-8.1547, 61.4431) (-8.6512, 60.9327) (-8.6512, 60.8306) knots 0 0 0 1 2 2 2
  spline S183 degree 2 poles (-8.6512, 60.8306) (-8.6512, 60.7666) (-8.5958, 60.7424) knots 0 0 0 1 1 1
  spline S184 degree 2 poles (-8.5958, 60.7424) (-8.5682, 60.7285) (-8.4938, 60.7216) knots 0 0 0 1 1 1
  spline S185 degree 2 poles (-8.4938, 60.7216) (-8.4384, 60.7164) (-8.4384, 60.6974) knots 0 0 0 1 1 1
  spline S186 degree 2 poles (-8.4384, 60.6974) (-8.4384, 60.668) (-8.5388, 60.668) knots 0 0 0 1 1 1
  spline S187 degree 2 poles (-8.5388, 60.668) (-8.7619, 60.668) (-8.7619, 60.8704) knots 0 0 0 1 1 1
  spline S188 degree 2 poles (-8.7619, 60.8704) (-8.7619, 60.9465) (-8.7048, 61.0694) knots 0 0 0 1 1 1
  spline S189 degree 2 poles (-8.0682, 61.3427) (-8.1097, 61.3237) (-8.1858, 61.2493) knots 0 0 0 1 1 1
  spline S190 degree 2 poles (-8.1858, 61.2493) (-8.2671, 61.1697) (-8.2671, 61.1386) knots 0 0 0 1 1 1
  line L46 (-8.2671, 61.1386) -> (-8.255, 61.1265)
  spline S191 degree 2 poles (-8.255, 61.1265) (-8.217, 61.1265) (-8.1477, 61.2147) knots 0 0 0 1 1 1
  spline S192 degree 2 poles (-8.1477, 61.2147) (-8.0907, 61.2908) (-8.0682, 61.3427) knots 0 0 0 1 1 1
  line L47 (-7.5093, 61.3306) -> (-7.8917, 61.0088)
  line L48 (-7.8917, 61.0088) -> (-8.1547, 60.8029)
  spline S193 degree 2 poles (-8.1547, 60.8029) (-8.3415, 60.6715) (-8.4609, 60.6715) knots 0 0 0 1 1 1
  spline S194 degree 2 poles (-8.4609, 60.6715) (-8.4782, 60.6715) (-8.4782, 60.6905) knots 0 0 0 1 1 1
  spline S195 degree 2 poles (-8.4782, 60.6905) (-8.4782, 60.7164) (-8.4488, 60.7234) knots 0 0 0 1 1 1
  spline S196 degree 2 poles (-8.4488, 60.7234) (-8.2619, 60.7683) (-7.9401, 61.0348) knots 0 0 0 1 1 1
  line L49 (-7.9401, 61.0348) -> (-7.5336, 61.3739)
  spline S197 degree 2 poles (-7.5336, 61.3739) (-7.3934, 61.4915) (-7.082, 61.8375) knots 0 0 0 1 1 1
  line L50 (-7.082, 61.8375) -> (-6.6824, 62.2943)
  spline S198 degree 2 poles (-6.6824, 62.2943) (-6.5872, 62.4067) (-6.5491, 62.4067) knots 0 0 0 1 1 1
  spline S199 degree 2 poles (-6.5491, 62.4067) (-6.499, 62.4067) (-6.499, 62.3566) knots 0 0 0 1 1 1
  spline S200 degree 2 poles (-6.499, 62.3566) (-6.499, 62.2943) (-6.6218, 62.142) knots 0 0 0 1 1 1
  line L51 (-6.6218, 62.142) -> (-6.7983, 61.9413)
  line L52 (-6.7983, 61.9413) -> (-7.3675, 61.2856)
  spline S201 degree 2 poles (-7.3675, 61.2856) (-7.1581, 61.4362) (-7.0595, 61.4362) knots 0 0 0 1 1 1
  spline S202 degree 2 poles (-7.0595, 61.4362) (-6.9436, 61.4362) (-6.9436, 61.322) knots 0 0 0 1 1 1
  spline S203 degree 2 poles (-6.9436, 61.322) (-6.9436, 61.1939) (-7.1685, 61.1022) knots 0 0 0 1 1 1
  spline S204 degree 2 poles (-7.1685, 61.1022) (-7.3519, 61.0279) (-7.5093, 61.0261) knots 0 0 0 1 1 1
  spline S205 degree 2 poles (-7.5093, 61.0261) (-7.4592, 60.905) (-7.3779, 60.751) knots 0 0 0 1 1 1
  spline S206 degree 2 poles (-7.3779, 60.751) (-7.3502, 60.7182) (-7.2896, 60.7182) knots 0 0 0 1 1 1
  spline S207 degree 2 poles (-7.2896, 60.7182) (-7.2689, 60.7182) (-7.2689, 60.6957) knots 0 0 0 1 1 1
  spline S208 degree 2 poles (-7.2689, 60.6957) (-7.2689, 60.6645) (-7.3796, 60.6645) knots 0 0 0 1 1 1
  spline S209 degree 2 poles (-7.3796, 60.6645) (-7.4349, 60.6645) (-7.473, 60.6922) knots 0 0 0 1 1 1
  spline S210 degree 2 poles (-7.473, 60.6922) (-7.5076, 60.7164) (-7.6287, 60.9742) knots 0 0 0 1 1 1
  line L53 (-7.6287, 60.9742) -> (-7.7723, 60.8029)
  spline S211 degree 2 poles (-7.7723, 60.8029) (-7.8917, 60.6628) (-7.9159, 60.6628) knots 0 0 0 1 1 1
  spline S212 degree 2 poles (-7.9159, 60.6628) (-7.9765, 60.6628) (-7.9765, 60.7337) knots 0 0 0 1 1 1
  spline S213 degree 2 poles (-7.9765, 60.7337) (-7.9765, 60.7753) (-7.7516, 61.0469) knots 0 0 0 1 1 1
  line L54 (-7.7516, 61.0469) -> (-7.5093, 61.3306)
  spline S214 degree 2 poles (-7.5526, 61.059) (-7.3398, 61.0867) (-7.063, 61.2666) (-7.063, 61.3306) knots 0 0 0 1 2 2 2
  spline S215 degree 2 poles (-7.063, 61.3306) (-7.063, 61.3635) (-7.1045, 61.3635) knots 0 0 0 1 1 1
  spline S216 degree 2 poles (-7.1045, 61.3635) (-7.2602, 61.3635) (-7.5526, 61.059) knots 0 0 0 1 1 1
  spline S217 degree 2 poles (-6.7585, 60.9016) (-6.8294, 60.8843) (-7.0266, 60.7701) knots 0 0 0 1 1 1
  spline S218 degree 2 poles (-7.0266, 60.7701) (-7.2014, 60.6715) (-7.2913, 60.6715) knots 0 0 0 1 1 1
  spline S219 degree 2 poles (-7.2913, 60.6715) (-7.3086, 60.6715) (-7.3086, 60.6905) knots 0 0 0 1 1 1
  spline S220 degree 2 poles (-7.3086, 60.6905) (-7.3086, 60.7182) (-7.2723, 60.7234) knots 0 0 0 1 1 1
  spline S221 degree 2 poles (-7.2723, 60.7234) (-7.1841, 60.7372) (-7.0266, 60.8289) knots 0 0 0 1 1 1
  spline S222 degree 2 poles (-7.0266, 60.8289) (-6.8519, 60.9275) (-6.7412, 60.9535) knots 0 0 0 1 1 1
  spline S223 degree 2 poles (-6.7412, 60.9535) (-6.6754, 61.1126) (-6.4695, 61.2874) knots 0 0 0 1 1 1
  spline S224 degree 2 poles (-6.4695, 61.2874) (-6.2516, 61.4742) (-6.0976, 61.4742) knots 0 0 0 1 1 1
  spline S225 degree 2 poles (-6.0976, 61.4742) (-5.9834, 61.4742) (-5.9834, 61.3773) knots 0 0 0 1 1 1
  spline S226 degree 2 poles (-5.9834, 61.3773) (-5.9834, 61.2493) (-6.2256, 61.0988) knots 0 0 0 1 1 1
  spline S227 degree 2 poles (-6.2256, 61.0988) (-6.4021, 60.9881) (-6.5872, 60.924) knots 0 0 0 1 1 1
  spline S228 degree 2 poles (-6.5872, 60.924) (-6.608, 60.8791) (-6.608, 60.8306) knots 0 0 0 1 1 1
  spline S229 degree 2 poles (-6.608, 60.8306) (-6.608, 60.7562) (-6.5561, 60.7337) knots 0 0 0 1 1 1
  spline S230 degree 2 poles (-6.5561, 60.7337) (-6.5301, 60.7251) (-6.4592, 60.7216) knots 0 0 0 1 1 1
  spline S231 degree 2 poles (-6.4592, 60.7216) (-6.4073, 60.7199) (-6.4073, 60.6957) knots 0 0 0 1 1 1
  spline S232 degree 2 poles (-6.4073, 60.6957) (-6.4073, 60.6593) (-6.5837, 60.6593) knots 0 0 0 1 1 1
  spline S233 degree 2 poles (-6.5837, 60.6593) (-6.7689, 60.6593) (-6.7689, 60.8202) knots 0 0 0 1 1 1
  spline S234 degree 2 poles (-6.7689, 60.8202) (-6.7689, 60.8566) (-6.7585, 60.9016) knots 0 0 0 1 1 1
  spline S235 degree 2 poles (-6.5716, 60.9829) (-6.4401, 61.0469) (-6.2931, 61.1576) knots 0 0 0 1 1 1
  spline S236 degree 2 poles (-6.2931, 61.1576) (-6.0993, 61.3012) (-6.0993, 61.386) knots 0 0 0 1 1 1
  spline S237 degree 2 poles (-6.0993, 61.386) (-6.0993, 61.4206) (-6.1304, 61.4206) knots 0 0 0 1 1 1
  spline S238 degree 2 poles (-6.1304, 61.4206) (-6.2239, 61.4206) (-6.383, 61.2493) knots 0 0 0 1 1 1
  spline S239 degree 2 poles (-6.383, 61.2493) (-6.5266, 61.0919) (-6.5716, 60.9829) knots 0 0 0 1 1 1
  spline S240 degree 2 poles (-5.6253, 61.3029) (-5.6322, 61.3497) (-5.6322, 61.36) knots 0 0 0 1 1 1
  spline S241 degree 2 poles (-5.6322, 61.36) (-5.6322, 61.3981) (-5.4488, 61.5625) (-5.4142, 61.5625) knots 0 0 0 1 2 2 2
  spline S242 degree 2 poles (-5.4142, 61.5625) (-5.3813, 61.5625) (-5.3813, 61.533) knots 0 0 0 1 1 1
  spline S243 degree 2 poles (-5.3813, 61.533) (-5.3813, 61.5071) (-5.4176, 61.4465) knots 0 0 0 1 1 1
  spline S244 degree 2 poles (-5.4176, 61.4465) (-5.255, 61.4465) (-5.255, 61.3185) knots 0 0 0 1 1 1
  spline S245 degree 2 poles (-5.255, 61.3185) (-5.255, 61.2182) (-5.6702, 60.7753) (-5.6702, 60.7476) knots 0 0 0 1 2 2 2
  spline S246 degree 2 poles (-5.6702, 60.7476) (-5.6702, 60.7234) (-5.6426, 60.7199) knots 0 0 0 1 1 1
  line L55 (-5.6426, 60.7199) -> (-5.5958, 60.7216)
  spline S247 degree 2 poles (-5.5958, 60.7216) (-5.5768, 60.7216) (-5.5768, 60.6974) knots 0 0 0 1 1 1
  spline S248 degree 2 poles (-5.5768, 60.6974) (-5.5768, 60.668) (-5.6599, 60.668) knots 0 0 0 1 1 1
  spline S249 degree 2 poles (-5.6599, 60.668) (-5.7654, 60.668) (-5.7654, 60.7614) knots 0 0 0 1 1 1
  spline S250 degree 2 poles (-5.7654, 60.7614) (-5.7654, 60.8548) (-5.6599, 60.9933) knots 0 0 0 1 1 1
  spline S251 degree 2 poles (-5.6599, 60.9933) (-5.5941, 61.0798) (-5.4661, 61.2095) knots 0 0 0 1 1 1
  spline S252 degree 2 poles (-5.4661, 61.2095) (-5.3606, 61.3133) (-5.3606, 61.3237) knots 0 0 0 1 1 1
  spline S253 degree 2 poles (-5.3606, 61.3237) (-5.3606, 61.3445) (-5.3848, 61.3445) knots 0 0 0 1 1 1
  spline S254 degree 2 poles (-5.3848, 61.3445) (-5.4055, 61.3445) (-5.5249, 61.3116) (-5.537, 61.3012) knots 0 0 0 1 2 2 2
  spline S255 degree 2 poles (-5.537, 61.3012) (-6.1997, 60.6715) (-6.4298, 60.6715) knots 0 0 0 1 1 1
  spline S256 degree 2 poles (-6.4298, 60.6715) (-6.4471, 60.6715) (-6.4471, 60.6905) knots 0 0 0 1 1 1
  spline S257 degree 2 poles (-6.4471, 60.6905) (-6.4471, 60.7164) (-6.409, 60.7234) knots 0 0 0 1 1 1
  spline S258 degree 2 poles (-6.409, 60.7234) (-6.3623, 60.732) (-6.2844, 60.7683) knots 0 0 0 1 1 1
  spline S259 degree 2 poles (-6.2844, 60.7683) (-6.1685, 60.8185) (-5.9401, 61.0106) knots 0 0 0 1 1 1
  spline S260 degree 2 poles (-5.9401, 61.0106) (-5.736, 61.1801) (-5.6253, 61.3029) knots 0 0 0 1 1 1
  line L56 (-4.6616, 61.3099) -> (-5.1166, 60.9327)
  spline S261 degree 2 poles (-5.1166, 60.9327) (-5.4609, 60.6715) (-5.5993, 60.6715) knots 0 0 0 1 1 1
  spline S262 degree 2 poles (-5.5993, 60.6715) (-5.6166, 60.6715) (-5.6166, 60.6905) knots 0 0 0 1 1 1
  spline S263 degree 2 poles (-5.6166, 60.6905) (-5.6166, 60.7164) (-5.5872, 60.7234) knots 0 0 0 1 1 1
  spline S264 degree 2 poles (-5.5872, 60.7234) (-5.4834, 60.7493) (-5.4263, 60.7804) knots 0 0 0 1 1 1
  spline S265 degree 2 poles (-5.4263, 60.7804) (-5.3363, 60.8272) (-5.0491, 61.0555) knots 0 0 0 1 1 1
  spline S266 degree 2 poles (-5.0491, 61.0555) (-4.9194, 61.1559) (-4.6754, 61.3773) knots 0 0 0 1 1 1
  spline S267 degree 2 poles (-4.6754, 61.3773) (-4.5837, 61.4725) (-4.5439, 61.4725) knots 0 0 0 1 1 1
  spline S268 degree 2 poles (-4.5439, 61.4725) (-4.4644, 61.4725) (-4.4644, 61.4206) knots 0 0 0 1 1 1
  spline S269 degree 2 poles (-4.4644, 61.4206) (-4.4644, 61.3548) (-4.6253, 61.149) knots 0 0 0 1 1 1
  spline S270 degree 2 poles (-4.6253, 61.149) (-4.3138, 61.4344) (-4.1962, 61.4344) knots 0 0 0 1 1 1
  spline S271 degree 2 poles (-4.1962, 61.4344) (-4.1564, 61.4344) (-4.0907, 61.3843) (-4.0907, 61.3462) knots 0 0 0 1 2 2 2
  spline S272 degree 2 poles (-4.0907, 61.3462) (-4.0907, 61.2891) (-4.1685, 61.1784) knots 0 0 0 1 1 1
  spline S273 degree 2 poles (-4.1685, 61.1784) (-3.8796, 61.4638) (-3.7135, 61.4638) knots 0 0 0 1 1 1
  spline S274 degree 2 poles (-3.7135, 61.4638) (-3.6183, 61.4638) (-3.6183, 61.386) knots 0 0 0 1 1 1
  spline S275 degree 2 poles (-3.6183, 61.386) (-3.6183, 61.2856) (-4.0872, 60.8047) (-4.0872, 60.7562) knots 0 0 0 1 2 2 2
  spline S276 degree 2 poles (-4.0872, 60.7562) (-4.0872, 60.7199) (-3.9868, 60.7182) (-3.9868, 60.6957) knots 0 0 0 1 2 2 2
  spline S277 degree 2 poles (-3.9868, 60.6957) (-3.9868, 60.668) (-4.0699, 60.668) knots 0 0 0 1 1 1
  spline S278 degree 2 poles (-4.0699, 60.668) (-4.1824, 60.668) (-4.1824, 60.7666) knots 0 0 0 1 1 1